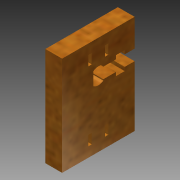
# Autodesk Inventor part: frame_y
Saved by Autodesk Inventor 2014 (Build 180170000, 170)
## iProperties
Created: 2015-01-04
Part Number: frame_y
Material: Generic
Document SubType Name: Modeling
Designer: cruiser
Density: 1 g/cm^3
Appearance: Yellow Pine - Solid Stained Light Low Gloss
Author: cruiser
Autodesk Inventor part; units mm, degrees
ref_plane "YZ Plane" through (0, 0, 0) normal (1, 0, 0) x (0, 1, 0)
ref_plane "XZ Plane" through (0, 0, 0) normal (0, 1, 0) x (-1, 0, 0)
ref_plane "XY Plane" through (0, 0, 0) normal (0, 0, 1) x (1, 0, 0)
sketch "Sketch1" plane through (0, 0, 0) normal (1, 0, 0) x (0, 1, 0)
  line L0 (0, 0) -> (-10.9877, 0)
  line L1 (-10.9877, 0) -> (-10.9877, -20)
  line L2 (-10.9877, -20) -> (0, -20)
  line L3 (0, -20) -> (0, 0)
  line L4 (0, 0) -> (10.9877, 0)
  line L5 (10.9877, 0) -> (10.9877, -20)
  line L6 (10.9877, -20) -> (0, -20)
  line L7 (-10.9877, 0) -> (10.9877, 0)
  line L8 (10.9877, 0) -> (10.9877, 10)
  line L9 (10.9877, 10) -> (-10.9877, 10)
  line L10 (-10.9877, 10) -> (-10.9877, 0)
  line L11 (-3, 7) -> (-2, 7)
  line L12 (-2, 7) -> (-2, 4)
  line L13 (-2, 4) -> (-3, 4)
  line L14 (-3, 4) -> (-3, 7)
  line L15 (3, 7) -> (2, 7)
  line L16 (2, 7) -> (2, 4)
  line L17 (2, 4) -> (3, 4)
  line L18 (3, 4) -> (3, 7)
  line L19 (-10.9877, -5) -> (10.9877, -5)
  line L20 (-3, -17) -> (-2, -17)
  line L21 (-2, -17) -> (-2, -14)
  line L22 (-2, -14) -> (-3, -14)
  line L23 (-3, -14) -> (-3, -17)
  line L24 (2, -14) -> (3, -14)
  line L25 (2, -17) -> (2, -14)
  line L26 (3, -17) -> (2, -17)
  line L27 (3, -14) -> (3, -17)
  arc A0 (1.5, 2) -> (0, 2.5) centre (0, 0) ccw
  line L28 (-1.5, -2) -> (1.5, -2)
  line L29 (1.5, -2) -> (1.5, 0)
  line L30 (1.5, 2) -> (-1.5, 2)
  line L31 (-1.5, 2) -> (-1.5, 0)
  line L32 (-1.5, -2) -> (1.5, 2) construction
  line L33 (1.5, -2) -> (-1.5, 2) construction
  arc A1 (2, 1.5) -> (1.5, 2) centre (0, 0) ccw
  arc A2 (0, -2.5) -> (1.5, -2) centre (0, 0) ccw
  arc A3 (-1.5, -2) -> (0, -2.5) centre (0, 0) ccw
  arc A4 (-1.5, 2) -> (-2, 1.5) centre (0, 0) ccw
  arc A5 (0, 2.5) -> (-1.5, 2) centre (0, 0) ccw
  line L34 (-1.5, 0) -> (-1.5, -2)
  line L35 (1.5, 0) -> (1.5, 2)
  dimension "d1" = 20
  dimension "d2" = 10
  dimension "d3" = 1
  dimension "d4" = 3
  dimension "d5" = 3
  dimension "d6" = 3
  dimension "d9" = 5
  dimension "d10" = 3
  constraints: 72 end point, 14 symmetric about line, 12 point on circle, 11 parallel, 8 point on line, 6 centre point, 6 perpendicular, 4 horizontal, 2 midpoint, 1 coincident, 1 collinear, 1 other
  measures "d1" distance of L4.end L5.end
  measures "d2" distance of L7.end L8.end
  measures "d3" distance of L12.end L13.end
  measures "d4" distance of L11.end L12.end
  measures "d5" distance between parallel lines of L3 L14
  measures "d6" distance between parallel lines of L9 L11
  measures "d9" diameter of A0
  measures "d10" distance of L30.start L30.end
extrude "Extrusion1" add sketch "Sketch1" along normal blind 5.08 contours L34 A3 L3 L19 L1 L0 | L0 L10 L9 L8 L4 L35 A0 A5 L31 | L4 L5 L19 L3 A2 L29 | L19 L3 L2 L1 | L19 L5 L6 L3
sketch "Sketch2" plane through (5.08, 0, 0) normal (1, 0, 0) x (0, 0, -1)
  line L0 (-2, 1.5) -> (2, 1.5) projected
  arc A0 (-2, 1.5) -> (-2, -1.5) centre (0, 0) ccw projected
  line L1 (20, 10.9877) -> (-10, 10.9877) projected
  line L2 (2.75, 5.3877) -> (-2.75, 5.3877)
  line L3 (-2.75, 5.3877) -> (-2.75, 7.9877)
  line L4 (-2.75, 7.9877) -> (2.75, 7.9877)
  line L5 (2.75, 7.9877) -> (2.75, 5.3877)
  line L6 (2.75, 5.3877) -> (-2.75, 7.9877) construction
  line L7 (-2.75, 5.3877) -> (2.75, 7.9877) construction
  line L8 (1.65, 1.5) -> (-1.65, 1.5)
  line L9 (-1.65, 1.5) -> (-1.65, 10.9877)
  line L10 (-1.65, 10.9877) -> (1.65, 10.9877)
  line L11 (1.65, 10.9877) -> (1.65, 1.5)
  line L12 (1.65, 1.5) -> (-1.65, 10.9877) construction
  line L13 (-1.65, 1.5) -> (1.65, 10.9877) construction
  line L14 (0, 0) -> (0, 10.9877)
  point P0 (0, 6.6877)
  point P1 (0, 6.2439)
  dimension "d11" = 0
  dimension "d12" = 3.3
  dimension "d13" = 0
  dimension "d14" = 2.6
  dimension "d15" = 5.5
  dimension "d16" = 3
  constraints: 26 end point, 4 midpoint, 4 parallel, 3 perpendicular, 3 point on line, 2 horizontal
  measures "d11" distance between parallel lines of L1 L10
  measures "d12" distance of L8.start L8.end
  measures "d13" distance between parallel lines of L0 L8
  measures "d14" distance of L2.end L3.end
  measures "d15" distance of L3.end L4.end
  measures "d16" distance between parallel lines of L1 L4
extrude "Extrusion2" cut sketch "Sketch2" against normal up to next
equation "\"d1\" = 0.5 * laser_body_length"
equation "\"d2\" = 0.25 * laser_body_length"
equation "\"d7\" = wood_thickness"
equation "\"wood_thickness\" = 5.08"
equation "\"m3_diameter\" = 3.15"
equation "\"m5_diameter\" = 5.25"
equation "\"stepper_screw_space\" = 35"
equation "\"stepper_shaft_diameter\" = 5"
equation "\"stepper_body_diameter\" = 28"
equation "\"laser_body_diameter\" = 12"
equation "\"laser_body_length\" = 40"
body "Solid1"
